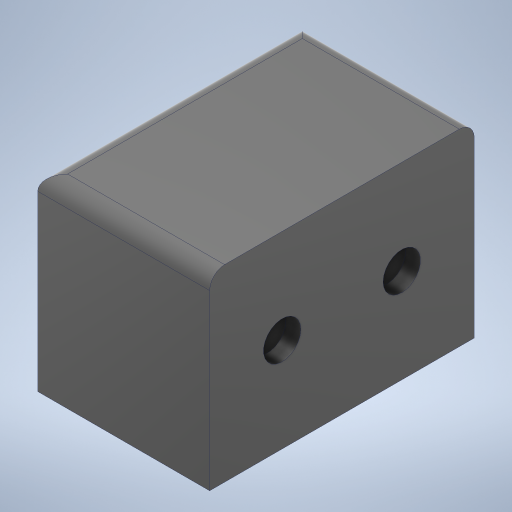
# Autodesk Inventor part: IR sensor
Saved by Autodesk Inventor 2024 (Build 280153000, 153)
## iProperties
Created: 2023-10-20
Part Number: IR sensor
Material: ABS Plastic
Document SubType Name: Modeling
Designer: kdcao
Density: 1.06 g/cm^3
Appearance: PTFE
Author: kdcao
Autodesk Inventor part; units mm, degrees
ref_plane "YZ Plane" through (0, 0, 0) normal (1, 0, 0) x (0, 1, 0)
ref_plane "XZ Plane" through (0, 0, 0) normal (0, 1, 0) x (-1, 0, 0)
sketch "Sketch2" plane through (0, 0, 0) normal (1, 0, 0) x (0, 1, 0)
  line L0 (-6.3, 8.85) -> (6.3, 8.85)
  line L1 (6.3, 8.85) -> (6.3, -8.85)
  line L2 (6.3, -8.85) -> (-6.3, -8.85)
  line L3 (-6.3, -8.85) -> (-6.3, 8.85)
  line L4 (-6.3, 8.85) -> (6.3, -8.85) construction
  line L5 (6.3, 8.85) -> (-6.3, -8.85) construction
  point P0 (0, 0)
  dimension "d0" = 17.7
  dimension "d1" = 12.6
  constraints: 12 end point, 2 midpoint, 2 parallel, 1 horizontal, 1 perpendicular
  measures "d0" distance of L0.end L1.end
  measures "d1" distance of L0.start L0.end
extrude "Extrusion1" add sketch "Sketch2" along normal blind 11.5
fillet "Fillet1" radius 1 3 edges at (5.75, 6.3, 8.85) (5.75, 6.3, -8.85) (0, 6.3, 0)
ref_plane "Work Plane1" through (0, -6.3, 0) normal (0, 0, 1) x (1, 0, 0)
sketch "Sketch3" plane through (11.5, 0, 0) normal (1, 0, 0) x (0, 0, -1)
  circle A0 centre (-4, 0) radius 1.25
  point P0 (0, 0)
  dimension "d5" = 2.5
  dimension "d6" = 4
  constraints: 1 centre point
  measures "d5" diameter of A0
  measures "d6" distance of point (0, 0) A0.centre
hole "Hole1" at (11.5, 0, 4) direction (-1, 0, 0) diameter 2.5 depth 1
mirror "Mirror1" about plane through (0, -6.3, 0) normal (0, 0, 1) of "Hole1"
body "Solid1"
